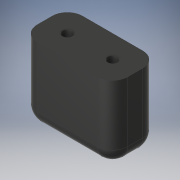
# Autodesk Inventor part: door_parts
Saved by Autodesk Inventor 2019 (Build 230136000, 136)
## iProperties
Created: 2019-07-22
Part Number: door_parts
Material: PAEK 樹脂
Document SubType Name: Modeling
Designer: gisen
Density: 1.32 g/cm^3
Appearance: 滑らか - 白
Author: gisen
Autodesk Inventor part; units mm, degrees
ref_plane "YZ Plane" through (0, 0, 0) normal (1, 0, 0) x (0, 1, 0)
ref_plane "XZ Plane" through (0, 0, 0) normal (0, 1, 0) x (-1, 0, 0)
ref_plane "XY Plane" through (0, 0, 0) normal (0, 0, 1) x (1, 0, 0)
sketch "スケッチ1" plane through (0, 0, 0) normal (0, 0, 1) x (1, 0, 0)
  line L0 (-26.4547, 10.8836) -> (3.5453, 10.8836)
  line L1 (3.5453, 10.8836) -> (3.5453, -14.1164)
  line L2 (3.5453, -14.1164) -> (-26.4547, -14.1164)
  line L3 (-26.4547, -14.1164) -> (-26.4547, 10.8836)
  point P0 (0, 0)
  dimension "d0" = 25
  dimension "d1" = 30
  constraints: 8 end point, 2 parallel, 1 horizontal, 1 perpendicular
  measures "d0" distance of L2.end L0.start
  measures "d1" distance of L0.start L0.end
extrude "押し出し1" add sketch "スケッチ1" along normal blind 15
sketch "スケッチ3" plane through (0, 0, 0) normal (0, 0, -1) x (-1, 0, 0)
  circle A0 centre (7.4547, -3.5864) radius 6
  line L0 (26.4547, 10.8836) -> (-3.5453, 10.8836) projected
  line L1 (-3.5453, 10.8836) -> (-3.5453, -14.1164) projected
  point P0 (0, 0)
  dimension "d7" = 12
  dimension "d8" = 14.47
  dimension "d9" = 11
  constraints: 1 centre point
  measures "d7" diameter of A0
  measures "d8" distance from line of L0 A0.centre
  measures "d9" distance from line of L1 A0.centre
extrude "押し出し2" cut sketch "スケッチ3" against normal blind 10
fillet "フィレット1" radius 5 8 edges at (3.5453, -14.1164, 7.5) (-11.4547, -14.1164, 15) (-11.4547, -14.1164, 0) (-26.4547, -1.6164, 15) (-26.4547, -14.1164, 7.5) (-26.4547, -1.6164, 0) (3.5453, -1.6164, 15) (3.5453, -1.6164, 0)
sketch "スケッチ4" plane through (-21.4547, 10.8836, 0) normal (0, 1, 0) x (1, 0, 0)
  arc A0 (25, -5) -> (20, 0) centre (20, -5) ccw projected
  line L0 (0, 0) -> (20, 0) projected
  arc A1 (0, 0) -> (-5, -5) centre (0, -5) ccw projected
  line L1 (-5, -5) -> (-5, -10) projected
  arc A2 (-5, -10) -> (0, -15) centre (0, -10) ccw projected
  line L2 (20, -15) -> (0, -15) projected
  arc A3 (20, -15) -> (25, -10) centre (20, -10) ccw projected
  line L3 (25, -5) -> (25, -10) projected
  circle A4 centre (17.5, -7.5) radius 1.65
  point P0 (21.4547, 0)
  dimension "d13" = 3.3
  dimension "d14" = 7.5
  dimension "d15" = 7.5
  constraints: 1 centre point
  measures "d13" diameter of A4
  measures "d14" distance from line of L3 A4.centre
  measures "d15" distance from line of L0 A4.centre
extrude "押し出し3" cut sketch "スケッチ4" against normal blind 7 contours A4
sketch "スケッチ5" plane through (-21.4547, 10.8836, 0) normal (0, 1, 0) x (1, 0, 0)
  circle A0 centre (17.5, -7.5) radius 1.65 projected
  circle A1 centre (2.5, -7.5) radius 1.65
  line L0 (-5, -5) -> (-5, -10) projected
  point P0 (21.4547, 0)
  dimension "d18" = 3.3
  dimension "d19" = 7.5
  constraints: 1 centre point
  measures "d18" diameter of A1
  measures "d19" distance from line of L0 A1.centre
extrude "押し出し4" cut sketch "スケッチ5" against normal blind 7 contours A1
